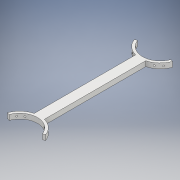
# Autodesk Inventor part: pendulum_arm
Saved by Autodesk Inventor 2017 (Build 210142000, 142)
## iProperties
Created: 2017-09-26
Part Number: pendulum_arm
Material: ABS Plastic
Document SubType Name: Modeling
Designer: Thoma
Density: 1.06 g/cm^3
Appearance: Smooth - White
Author: Thoma
Autodesk Inventor part; units mm, degrees
ref_plane "YZ Plane" through (0, 0, 0) normal (1, 0, 0) x (0, 1, 0)
ref_plane "XZ Plane" through (0, 0, 0) normal (0, 1, 0) x (-1, 0, 0)
ref_plane "XY Plane" through (0, 0, 0) normal (0, 0, 1) x (1, 0, 0)
sketch "Sketch1" plane through (0, 0, 0) normal (0, 0, 1) x (1, 0, 0)
  line L0 (0, 0) -> (-20, 0)
  line L1 (-20, 0) -> (-20, 200)
  line L2 (-20, 200) -> (0, 200)
  line L3 (0, 200) -> (0, 0)
  arc A0 (22.8892, -26.7591) -> (-42.8892, -26.7591) centre (-10, -38.7298) ccw
  line L4 (-42.8892, -26.7591) -> (-47.5877, -25.049)
  line L5 (-10, -38.7298) -> (30, -38.7298) construction
  line L6 (22.8892, -26.7591) -> (27.5877, -25.049)
  arc A1 (27.5877, -25.049) -> (0, 0) centre (-10, -38.7298) ccw
  arc A2 (-20, 0) -> (-47.5877, -25.049) centre (-10, -38.7298) ccw
  line L7 (-20, 100) -> (0, 100) construction
  line L8 (0, 200) -> (-20, 200)
  arc A3 (-42.8892, 226.7591) -> (22.8892, 226.7591) centre (-10, 238.7298) ccw
  line L9 (-42.8892, 226.7591) -> (-47.5877, 225.049)
  line L10 (-10, 238.7298) -> (30, 238.7298) construction
  line L11 (22.8892, 226.7591) -> (27.5877, 225.049)
  arc A4 (0, 200) -> (27.5877, 225.049) centre (-10, 238.7298) ccw
  arc A5 (-47.5877, 225.049) -> (-20, 200) centre (-10, 238.7298) ccw
  dimension "d0" = 20
  dimension "d3" = 70
  dimension "d4" = 160
  dimension "d5" = 200
  constraints: 24 end point, 12 point on circle, 6 centre point, 6 symmetric about line, 2 horizontal, 2 midpoint, 2 parallel, 1 perpendicular, 3 other
  measures "d0" distance of L1.end L2.end
  measures "d3" diameter of A0
  measures "d4" angle of L5 L4
  measures "d5" distance of L1.end L0.end
extrude "Extrusion1" add sketch "Sketch1" along normal blind 10
sketch "Sketch2" plane through (0, 0, 10) normal (0, 0, 1) x (1, 0, 0)
  arc A0 (-20, 0) -> (-47.5877, -25.049) centre (-10, -38.7298) ccw projected
  line L0 (-47.5877, -25.049) -> (-42.8892, -26.7591) projected
  arc A1 (22.8892, -26.7591) -> (-42.8892, -26.7591) centre (-10, -38.7298) ccw projected
  line L1 (22.8892, -26.7591) -> (27.5877, -25.049) projected
  arc A2 (27.5877, -25.049) -> (0, 0) centre (-10, -38.7298) ccw projected
  line L2 (0, 0) -> (0, 200) projected
  arc A3 (0, 200) -> (27.5877, 225.049) centre (-10, 238.7298) ccw projected
  line L3 (27.5877, 225.049) -> (22.8892, 226.7591) projected
  arc A4 (-42.8892, 226.7591) -> (22.8892, 226.7591) centre (-10, 238.7298) ccw projected
  line L4 (-42.8892, 226.7591) -> (-47.5877, 225.049) projected
  arc A5 (-47.5877, 225.049) -> (-20, 200) centre (-10, 238.7298) ccw projected
  line L5 (-20, 200) -> (-20, 0) projected
  arc A6 (27.5877, -25.049) -> (0, 0) centre (-10, -38.7298) ccw construction
  line L6 (-10, -38.7298) -> (-10, 1.2702) construction
  line L7 (-10, -38.7298) -> (11.6566, -5.0996) construction
  line L8 (-10, -38.7298) -> (30, -38.7298) construction
  line L9 (-10, -38.7298) -> (21.3911, -13.9387) construction
  line L10 (-10, -38.7298) -> (30, -38.7298) construction
  line L11 (-10, -38.7298) -> (-31.6566, -5.0996) construction
  line L12 (-10, -38.7298) -> (-41.3911, -13.9387) construction
  line L13 (0, 0) -> (0, 200) construction
  line L14 (0, 100) -> (30, 100) construction
  line L15 (0, 100) -> (-49.9249, 100) construction
  line L16 (-10, 238.7298) -> (11.6566, 205.0996) construction
  line L17 (-10, 238.7298) -> (21.3911, 213.9387) construction
  line L18 (-10, 238.7298) -> (-41.3911, 213.9387) construction
  line L19 (-10, 238.7298) -> (-31.6566, 205.0996) construction
  dimension "d8" = 57.22
  dimension "d9" = 38.3
  constraints: 26 end point, 7 symmetric about line, 4 horizontal, 2 equal length, 2 point on circle, 1 midpoint, 1 vertical
  measures "d8" angle of L8 L7
  measures "d9" angle of L10 L9
ref_plane "Work Plane1" through (21.3911, -13.9387, 10) normal (0.7847764, 0.619779, 0) x (-0.619779, 0.7847764, 0)
ref_plane "Work Plane2" through (11.6566, -5.0996, 10) normal (0.5414148, 0.8407556, 0) x (-0.8407556, 0.5414148, 0)
ref_plane "Work Plane3" through (-31.6566, -5.0996, 10) normal (-0.5414148, 0.8407556, 0) x (-0.8407556, -0.5414148, 0)
ref_plane "Work Plane4" through (-41.3911, -13.9387, 10) normal (-0.7847764, 0.619779, 0) x (-0.619779, -0.7847764, 0)
ref_plane "Work Plane5" through (-31.6566, 205.0996, 10) normal (-0.5414148, -0.8407556, 0) x (0.8407556, -0.5414148, 0)
ref_plane "Work Plane6" through (-41.3911, 213.9387, 10) normal (-0.7847764, -0.619779, 0) x (0.619779, -0.7847764, 0)
ref_plane "Work Plane7" through (11.6566, 205.0996, 10) normal (0.5414148, -0.8407556, 0) x (0.8407556, 0.5414148, 0)
ref_plane "Work Plane8" through (21.3911, 213.9387, 10) normal (0.7847764, -0.619779, 0) x (0.619779, 0.7847764, 0)
sketch "Sketch3" plane through (21.3911, -13.9387, 10) normal (0.7847764, 0.619779, 0) x (-0.619779, 0.7847764, 0)
  line L0 (24.1965, -10) -> (-12.5597, -10) construction
  point P0 (0, 0)
  point P1 (0, -5)
  dimension "d10" = 5
  measures "d10" distance from line of L0 point (0, -5)
sketch "Sketch4" plane through (11.6566, -5.0996, 10) normal (0.5414148, 0.8407556, 0) x (-0.8407556, 0.5414148, 0)
  line L0 (12.5613, -10) -> (-24.1951, -10) projected
  point P0 (0, 0)
  point P1 (0, -5)
  dimension "d11" = 5
  measures "d11" distance from line of L0 point (0, -5)
sketch "Sketch5" plane through (-31.6566, -5.0996, 10) normal (-0.5414148, 0.8407556, 0) x (-0.8407556, -0.5414148, 0)
  point P0 (-29.3765, -10)
  point P1 (0, 0)
  point P2 (0, -5)
  dimension "d12" = 5
  measures "d12" distance of point (0, 0) point (0, -5)
sketch "Sketch6" plane through (-41.3911, -13.9387, 10) normal (-0.7847764, 0.619779, 0) x (-0.619779, -0.7847764, 0)
  point P0 (-36.592, -10)
  point P1 (0, 0)
  point P2 (0, -5)
  dimension "d13" = 5
  measures "d13" distance of point (0, 0) point (0, -5)
sketch "Sketch8" plane through (-41.3911, 213.9387, 10) normal (-0.7847764, -0.619779, 0) x (0.619779, -0.7847764, 0)
  point P0 (193.5473, -10)
  point P1 (0, 0)
  point P2 (0, -5)
  dimension "d14" = 5
  measures "d14" distance of point (0, 0) point (0, -5)
sketch "Sketch9" plane through (-31.6566, 205.0996, 10) normal (-0.5414148, -0.8407556, 0) x (0.8407556, -0.5414148, 0)
  point P0 (137.6594, -10)
  point P1 (0, 0)
  point P2 (0, -5)
  dimension "d15" = 5
  measures "d15" distance of point (0, 0) point (0, -5)
sketch "Sketch10" plane through (21.3911, 213.9387, 10) normal (0.7847764, -0.619779, 0) x (0.619779, 0.7847764, 0)
  point P0 (-181.1517, -10)
  point P1 (0, 0)
  point P2 (0, -5)
  dimension "d16" = 5
  measures "d16" distance of point (0, 0) point (0, -5)
sketch "Sketch11" plane through (11.6566, 205.0996, 10) normal (0.5414148, -0.8407556, 0) x (0.8407556, 0.5414148, 0)
  point P0 (-120.8443, -10)
  point P1 (0, 0)
  point P2 (0, -5)
  dimension "d17" = 5
  measures "d17" distance of point (0, -5) point (0, 0)
hole "Hole1" at (21.3911, 213.9387, 5) direction (-0.7847764, 0.619779, 0) diameter 3 depth 8 tip angle 118
hole "Hole2" at (11.6566, 205.0996, 5) direction (-0.5414148, 0.8407556, 0) diameter 3 depth 8 tip angle 118
hole "Hole3" at (-31.6566, 205.0996, 5) direction (0.5414148, 0.8407556, 0) diameter 3 depth 8 tip angle 118
hole "Hole4" at (-41.3911, 213.9387, 5) direction (0.7847764, 0.619779, 0) diameter 3 depth 8 tip angle 118
hole "Hole5" at (-31.6566, -5.0996, 5) direction (0.5414148, -0.8407556, 0) diameter 3 depth 8 tip angle 118
hole "Hole6" at (-41.3911, -13.9387, 5) direction (0.7847764, -0.619779, 0) diameter 3 depth 8 tip angle 118
hole "Hole7" at (11.6566, -5.0996, 5) direction (-0.5414148, -0.8407556, 0) diameter 3 depth 8 tip angle 118
hole "Hole8" at (21.3911, -13.9387, 5) direction (-0.7847764, -0.619779, 0) diameter 3 depth 8 tip angle 118
body "Solid1"
